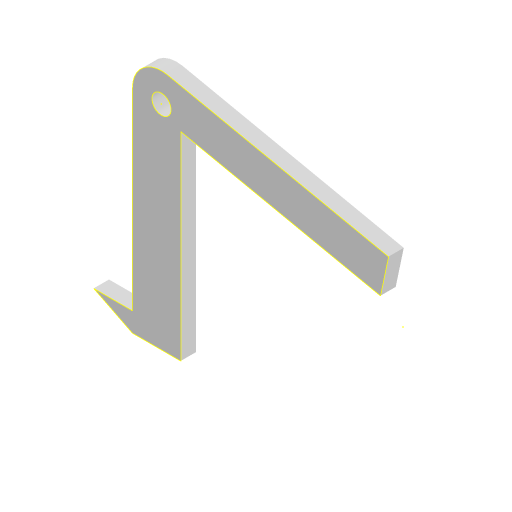
# Autodesk Inventor part: Lever
Saved by Autodesk Inventor 2023 (Build 270158000, 158)
## iProperties
Created: 2022-10-25
Part Number: Lever
Material: Generic
Document SubType Name: Modeling
Designer: deli
Density: 1 g/cm^3
Appearance: Default
Author: deli
Autodesk Inventor part; units mm, degrees
ref_plane "YZ Plane" through (0, 0, 0) normal (1, 0, 0) x (0, 1, 0)
ref_plane "XZ Plane" through (0, 0, 0) normal (0, 1, 0) x (-1, 0, 0)
ref_plane "XY Plane" through (0, 0, 0) normal (0, 0, 1) x (1, 0, 0)
sketch "Sketch1" plane through (0, 0, 0) normal (0, 0, 1) x (1, 0, 0)
  line L0 (-55.9809, 14.9531) -> (-55.9809, -25.0469)
  line L1 (-55.9809, -25.0469) -> (-63.9809, -25.0469)
  line L2 (-63.9809, -25.0469) -> (-55.9809, -29.0469)
  line L3 (-55.9809, -29.0469) -> (-45.9809, -29.0469)
  line L4 (-45.9809, -29.0469) -> (-45.9809, 12.0581)
  line L5 (-45.9809, 12.0581) -> (-4.6837, 3.2802)
  line L6 (-4.6837, 3.2802) -> (-3.0205, 11.1053)
  line L7 (-3.0205, 11.1053) -> (-48.7334, 20.8219)
  arc A0 (-48.7334, 20.8219) -> (-55.9809, 14.9531) centre (-49.9809, 14.9531) ccw
  circle A1 centre (-49.9809, 14.9531) radius 2
  point P0 (0, 0)
  dimension "d0" = 4
  dimension "d1" = 6
  dimension "d2" = 10
  dimension "d3" = 4
  dimension "d4" = 8
  dimension "d5" = 40
  dimension "d6" = 8
  dimension "d7" = 78
  dimension "d10" = 10
  constraints: 16 end point, 3 perpendicular, 2 centre point, 2 parallel, 2 point on circle, 2 tangent, 1 coincident, 1 vertical
  measures "d0" diameter of A1
  measures "d1" radius of A0
  measures "d2" distance between parallel lines of L4 L0
  measures "d3" distance between parallel lines of L3 L1
  measures "d4" distance of L0.end L1.end
  measures "d5" distance of L0.start L0.end
  measures "d6" distance between parallel lines of L7 L5
  measures "d7" angle of L5 L4
  measures "d10" distance of L2.end L3.end
extrude "Extrusion1" add sketch "Sketch1" along normal blind 3.175
sketch "Sketch2" plane through (0, 0, 3.175) normal (0, 0, 1) x (1, 0, 0)
  line L0 (-55.9809, -25.0469) -> (-63.9809, -25.0469) projected
  line L1 (-63.9809, -25.0469) -> (-55.9809, -29.0469) projected
  line L2 (-55.9809, -29.0469) -> (-45.9809, -29.0469) projected
  line L3 (-45.9809, -29.0469) -> (-45.9809, 12.0581) projected
  line L4 (-45.9809, 12.0581) -> (-4.6837, 3.2802) projected
  line L5 (-4.6837, 3.2802) -> (-3.0205, 11.1053) projected
  line L6 (-3.0205, 11.1053) -> (-48.7334, 20.8219) projected
  arc A0 (-48.7334, 20.8219) -> (-55.9809, 14.9531) centre (-49.9809, 14.9531) ccw projected
  line L7 (-55.9809, 14.9531) -> (-55.9809, -25.0469) projected
  circle A1 centre (-49.9809, 14.9531) radius 2 projected
  point P0 (0, 0)
equation "\"d10\" = d2"
body "Solid1"
